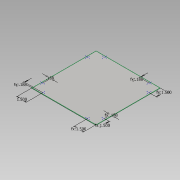
# Autodesk Inventor part: XY Carriage
Saved by Autodesk Inventor 2,016 (Build 200138000, 138)
## iProperties
Created: 2017-05-15
Part Number: XY Carriage
Material: Generic
Document SubType Name: Modeling
Designer: 31745
Density: 1 g/cm^3
Appearance: Default
Author: 31745
Autodesk Inventor part; units mm, degrees
ref_plane "YZ Plane" through (0, 0, 0) normal (1, 0, 0) x (0, 1, 0)
ref_plane "XZ Plane" through (0, 0, 0) normal (0, 1, 0) x (-1, 0, 0)
ref_plane "XY Plane" through (0, 0, 0) normal (0, 0, 1) x (1, 0, 0)
sketch "Sketch1" plane through (0, 0, 0) normal (0, 1, 0) x (-1, 0, 0)
  line L0 (0, 0) -> (-254, 0)
  line L1 (-254, 0) -> (-254, -254)
  line L2 (-254, -254) -> (0, -254)
  line L3 (0, -254) -> (0, 0)
  dimension "d0" = 254
  dimension "d1" = 254
  constraints: 8 end point, 2 parallel, 1 horizontal, 1 perpendicular
  measures "d0" distance of L2.end L1.end
  measures "d1" distance of L1.end L0.end
extrude "Extrusion1" add sketch "Sketch1" along normal blind 2.286
sketch "Sketch2" plane through (0, 2.286, 0) normal (0, 1, 0) x (1, 0, 0)
  line L0 (0, 0) -> (254, 0) projected
  line L1 (254, 0) -> (254, 254) projected
  line L2 (254, 254) -> (0, 254) projected
  line L3 (0, 254) -> (0, 0) projected
  point P0 (38.1, 4.7625)
  point P1 (215.9, 4.7625)
  point P2 (4.7625, 38.1)
  point P3 (4.7625, 215.9)
  point P4 (38.1, 249.2375)
  point P5 (215.9, 249.2375)
  point P6 (249.2375, 215.9)
  point P7 (249.2375, 38.1)
  dimension "d4" = 38.1
  dimension "d5" = 38.1
  dimension "d6" = 38.1
  dimension "d7" = 38.1
  dimension "d8" = 4.7625
  dimension "d9" = 4.7625
  dimension "d10" = 4.7625
  dimension "d11" = 4.7625
  constraints: 4 horizontal alignment, 4 vertical alignment
  measures "d4" distance from line of L3 point (38.1, 4.763)
  measures "d5" distance from line of L1 point (215.9, 4.763)
  measures "d6" distance from line of L0 point (249.237, 38.1)
  measures "d7" distance from line of L2 point (249.237, 215.9)
  measures "d8" distance from line of L3 point (4.762, 38.1)
  measures "d9" distance from line of L0 point (38.1, 4.763)
  measures "d10" distance from line of L1 point (249.237, 38.1)
  measures "d11" distance from line of L2 point (215.9, 249.237)
equation "\"d0\" = d1"
equation "\"d5\" = d4"
equation "\"d6\" = d5"
equation "\"d7\" = d6"
equation "\"d9\" = d8"
equation "\"d10\" = d9"
equation "\"d11\" = d8"
body "Solid1"
